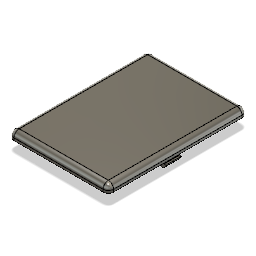
Slide Case (Autodesk Fusion 360 archive; units mm, degrees)
design "Sensor Lid"
Autodesk Fusion 360 part; units mm, degrees
box "BoxPrimitive1" add length 53 width 38 height 3 placed x (0, 0, 1) y (1, 0, 0) z (0, 1, 0) at (-3, 17, -2) makes body 1
fillet "Fillet1" radius 2 8 edges at (35, 18.5, -2) (35, 20, 24.5) (16, 20, -2) (-3, 18.5, -2) (-3, 20, 24.5) (16, 20, 51) (35, 18.5, 51) (-3, 18.5, 51) on bodies 1
shell "Shell1" thickness 2 removed faces 1 at (9.6667, 17, 32.6667) on bodies 1
fillet "Fillet2" radius 2 4 edges at (-1, 17.5, 49) (33, 17.5, 0) (-1, 17.5, 0) (33, 17.5, 49) on bodies 1
sketch "Sketch1" plane through (0, 18, 0) normal (0, -1, 0) x (1, 0, 0)
  arc A0 (33, 47) -> (31, 49) centre (31, 47) ccw
  line L0 (31, 49) -> (1, 49)
  arc A1 (1, 49) -> (-1, 47) centre (1, 47) ccw
  line L1 (-1, 47) -> (-1, 2)
  arc A2 (-1, 2) -> (1, 0) centre (1, 2) ccw
  line L2 (1, 0) -> (31, 0)
  arc A3 (31, 0) -> (33, 2) centre (31, 2) ccw
  line L3 (33, 2) -> (33, 47)
  line L4 (-1, 2) -> (1, 2)
  line L5 (1, 2) -> (1, 0)
  dimension "d3" = 2
extrude "Extrude1" add sketch "Sketch1" along normal blind 2 separate body contours A2 L4 L5 makes body 2
ref_plane "WorkPlane3" through (16, 17.5, 24.5) normal (1, 0, 0) x (0, 1, 0)
ref_plane "WorkPlane5" through (16, 17.5, 24.5) normal (0, 0, -1) x (0, 1, 0)
mirror "Mirror1" about plane through (16, 17.5, 24.5) normal (1, 0, 0) of bodies 2 makes body 3
mirror "Mirror2" about plane through (16, 17.5, 24.5) normal (0, 0, -1) of bodies 3 2 makes body 4 at (32.9436, 16.6667, 47.4715) makes body 5 at (-0.9436, 16.6667, 47.4715)
sketch "Sketch2" plane through (16.5, 17.5, 24.5) normal (0, 0, -1) x (1, 0, 0)
  line L0 (-17.5, -0.5) -> (16.5, -0.5)
  line L1 (15, -0.5) -> (15, 4.5)
  line L2 (17, 3.5) -> (16, 4.5)
  line L3 (17, 3.5) -> (17, 3)
  line L4 (16, 4.5) -> (15, 4.5)
  line L5 (15, -0.5) -> (16.5, -0.5)
  line L6 (16.5, -0.5) -> (16.5, 0.5)
  line L7 (16.5, 0.5) -> (16.3, 0.5)
  line L8 (16.3, 0.5) -> (16.3, 3)
  line L9 (17, 3) -> (16.3, 3)
  dimension "d14" = 0.5
  dimension "d16" = 5
  dimension "d23" = 0.2
  dimension "d24" = 1
  dimension "d25" = 1
  dimension "d26" = 1.5
  dimension "d27" = 1
  measures "d16" distance of L0 L4
  measures "d24" distance of L3
  measures "d27" distance of L4
extrude "Extrude2" add sketch "Sketch2" along normal mid plane 6 separate body makes body 6
mirror "Mirror3" about plane through (16, 17.5, 24.5) normal (1, 0, 0) of bodies 6 makes body 7
fillet "Fillet3" radius 2 1 edges at (-0.8, 17, 24.5) on bodies 7
fillet "Fillet4" radius 2 1 edges at (32.8, 17, 24.5) on bodies 6
combine "Combine1" operation add target body 7 tool bodies 6 1
fillet "Fillet5" radius 1 2 edges at (0.5, 18, 24.5) (31.5, 18, 24.5) on bodies 7
fillet "Fillet6" radius 1 4 edges at (0.25, 18, 27.5) (31.75, 18, 27.5) (31.75, 18, 21.5) (0.25, 18, 21.5) on bodies 7

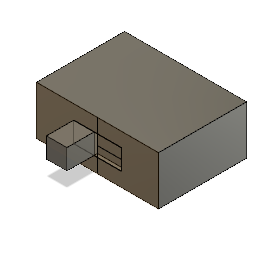
design "Switch"
Autodesk Fusion 360 part; units mm, degrees
sketch "Sketch1" plane through (0, 0, 0) normal (0, 1, 0) x (1, 0, 0)
box "BoxPrimitive1" add length 6.5 width 9 height 3.6 placed x (0, 0, 1) y (1, 0, 0) z (0, 1, 0) at (0, 0, 0)
sketch "Sketch2" plane through (0, 0, 6.5) normal (0, 0, 1) x (1, 0, 0)
  line L0 (0, 3.6) -> (0, 0)
  line L1 (0, 0) -> (9, 0)
  line L2 (9, 0) -> (9, 3.6)
  line L3 (9, 3.6) -> (0, 3.6)
  line L4 (4.5, 3.6) -> (4.5, 0)
  line L5 (4.5, 1.8) -> (6.25, 1.8)
  line L6 (6.25, 1.8) -> (6.25, 1.05)
  line L7 (6.25, 1.05) -> (2.75, 1.05)
  line L8 (2.75, 1.05) -> (2.75, 2.55)
  line L9 (2.75, 2.55) -> (6.25, 2.55)
  line L10 (6.25, 2.55) -> (6.25, 1.8)
  line L11 (2.75, 2.55) -> (4.25, 2.55)
  line L12 (4.25, 2.55) -> (4.25, 1.05)
  dimension "d6" = 1.75
  dimension "d7" = 0.75
  dimension "d8" = 3.5
  dimension "d9" = 1.5
  dimension "d10" = 3.5
  dimension "d11" = 1.5
extrude "Extrude1" add sketch "Sketch2" along normal blind 2 contours L7 L8 L9 L11 L12
extrude "Extrude2" cut sketch "Sketch2" against normal blind 0.25 contours L4 L5 L9 L10 | L4 L7 L9 L12 | L4 L5 L6 L7

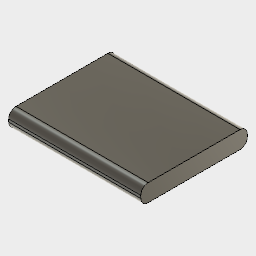
design "1578 500mAh battery"
Autodesk Fusion 360 part; units mm, degrees
sketch "Sketch1" plane through (0, 0, 0) normal (0, 0, 1) x (1, 0, 0)
  line L0 (0, 0) -> (36, 0)
  line L1 (36, 0) -> (36, 29)
  line L2 (36, 29) -> (0, 29)
  line L3 (0, 29) -> (0, 0)
  dimension "d1" = 36
  dimension "d2" = 29
  measures "d1" distance of L1.end L2.end
  measures "d2" distance of L0.start L2.end
extrude "Extrude1" add sketch "Sketch1" along normal blind 4.75
fillet "Fillet1" radius 2 4 edges at (18, 0, 4.75) (18, 0, 0) (18, 29, 4.75) (18, 29, 0)
